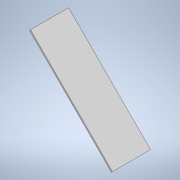
# Autodesk Inventor part: BeamSplitter
Saved by Autodesk Inventor 2022.2 (Build 262287010, 287A)
## iProperties
Created: 2022-03-22
Part Number: BeamSplitter
Material: Genérico
Document SubType Name: Modeling
Designer: mabel
Density: 1 g/cm^3
Appearance: Valor por defecto
Author: mabel
Autodesk Inventor part; units mm, degrees
ref_plane "YZ Plane" through (0, 0, 0) normal (1, 0, 0) x (0, 1, 0)
ref_plane "XZ Plane" through (0, 0, 0) normal (0, 1, 0) x (-1, 0, 0)
ref_plane "Plano de trabajo1" through (217.2201, -92.3211, 0) normal (0.7071, 0.7071, 0) x (0, 0, 1)
sketch "Boceto3" plane through (217.2201, -92.3211, 0) normal (0.7071, 0.7071, 0) x (0, 0, 1)
  line L0 (-11.614, 49.5404) -> (13.386, 49.5404)
  line L1 (13.386, 49.5404) -> (13.386, -26.4596)
  line L2 (13.386, -26.4596) -> (-11.614, -26.4596)
  line L3 (-11.614, -26.4596) -> (-11.614, 49.5404)
  line L4 (-11.614, 49.5404) -> (13.386, -26.4596) construction
  line L5 (13.386, 49.5404) -> (-11.614, -26.4596) construction
  point P0 (0, -218.8787)
  point P1 (0, 0)
  dimension "d10" = 25
  dimension "d11" = 76
  constraints: 12 end point, 2 parallel, 1 horizontal, 1 perpendicular
  measures "d10" distance of L1.end L2.end
  measures "d11" distance of L0.end L1.end
extrude "Extrusión3" add sketch "Boceto3" along normal blind 1
